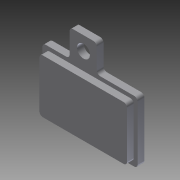
# Autodesk Inventor part: lid
Saved by Autodesk Inventor 2011 (Build 150239000, 239)
## iProperties
Created: 2011-02-17
Part Number: lid
Document SubType Name: Modeling
Designer: labuser
Density: 1 g/cm^3
Author: labuser
Autodesk Inventor part; units mm, degrees
ref_plane "YZ Plane" through (0, 0, 0) normal (1, 0, 0) x (0, 1, 0)
ref_plane "XZ Plane" through (0, 0, 0) normal (0, 1, 0) x (-1, 0, 0)
ref_plane "XY Plane" through (0, 0, 0) normal (0, 0, 1) x (1, 0, 0)
sketch "Sketch1" plane through (0, 0, 0) normal (0, 0, 1) x (1, 0, 0)
  line L0 (0, 0) -> (14, 0)
  line L1 (14, 0) -> (14, 9)
  line L2 (14, 9) -> (0, 9)
  line L3 (0, 9) -> (0, 0)
  dimension "d0" = 14
  dimension "d1" = 9
  constraints: 8 end point, 2 parallel, 1 horizontal, 1 perpendicular
  measures "d0" distance of L2.end L1.end
  measures "d1" distance of L1.end L0.end
extrude "Extrusion1" add sketch "Sketch1" along normal blind 2
sketch "Sketch2" plane through (0, 0, 2) normal (0, 0, 1) x (1, 0, 0)
  line L0 (0, 0) -> (0, 9) projected
  line L1 (14, 0) -> (0, 0) projected
  line L2 (14, 9) -> (14, 0) projected
  line L3 (0, 9) -> (14, 9) projected
  line L4 (0.5635, 8.4365) -> (0.5635, 0.5635)
  line L5 (0.5635, 0.5635) -> (13.4365, 0.5635)
  line L6 (13.4365, 0.5635) -> (13.4365, 8.4365)
  line L7 (13.4365, 8.4365) -> (0.5635, 8.4365)
  dimension "d4" = 0.5635
  constraints: 8 end point, 3 other
  measures "d4" distance between parallel lines of L0 L4
extrude "Extrusion2" cut sketch "Sketch2" against normal blind 1
sketch "Sketch3" plane through (0, 9, 0) normal (0, 1, 0) x (1, 0, 0)
  line L0 (0, -1) -> (14, -1) projected
  line L1 (14, 0) -> (0, 0) projected
  line L2 (0, 0) -> (0, -1) projected
  line L3 (4, 0) -> (8, 0)
  line L4 (8, 0) -> (8, -1)
  line L5 (8, -1) -> (4, -1)
  line L6 (4, -1) -> (4, 0)
  dimension "d7" = 4
  dimension "d8" = 4
  constraints: 8 end point, 2 parallel, 2 point on line, 1 horizontal, 1 perpendicular
  measures "d7" distance of L4.end L5.end
  measures "d8" distance between parallel lines of L6 L2
extrude "Extrusion3" add sketch "Sketch3" along normal blind 4 contours L6 L1 L4 L0
sketch "Sketch4" plane through (0, 0, 1) normal (0, 0, 1) x (1, 0, 0)
  line L0 (8, 13) -> (4, 13) projected
  line L1 (4, 9) -> (4, 13) projected
  line L2 (0, 0) -> (0, 9) projected
  line L3 (4, 11) -> (8.8648, 11) construction
  line L4 (6, 13) -> (6, 6.8956) construction
  point P0 (6.0394, 10.9642)
  constraints: 4 end point, 2 midpoint, 2 perpendicular
hole "Hole1" at (6.0394, 10.9642, 1) direction (0, 0, -1) diameter 1.905 end through all
fillet "Fillet1" radius 0.5 12 edges at (0.5635, 0.5635, 1.5) (0, 0, 0.5) (0.5635, 8.4365, 1.5) (0, 9, 0.5) (13.4365, 0.5635, 1.5) (14, 0, 0.5) (13.4365, 8.4365, 1.5) (14, 9, 0.5) (8, 9, 0.5) (4, 9, 0.5) (4, 13, 0.5) (8, 13, 0.5)
body "Solid1"
